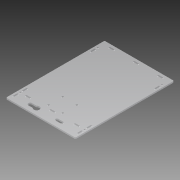
# Autodesk Inventor part: plastic_part_1
Saved by Autodesk Inventor 2013 (Build 170138000, 138)
## iProperties
Shininess: 20.0
Created: 2013-02-12
Part Number: plastic_part_1
Document SubType Name: Modeling
Designer: Noa Izumi
Material: Default
Density: 1 g/cm^3
Density: 0.0
Volumn: 0.0
Area: 0.0
PropertySet Name: Model Information
Control State: 0
Master: False
Checked Out: False
Author: Noa Izumi
Autodesk Inventor part; units mm, degrees
ref_plane "YZ Plane" through (0, 0, 0) normal (1, 0, 0) x (0, 1, 0)
ref_plane "XZ Plane" through (0, 0, 0) normal (0, 1, 0) x (-1, 0, 0)
ref_plane "XY Plane" through (0, 0, 0) normal (0, 0, 1) x (1, 0, 0)
sketch "Sketch1" plane through (0, 0, 0) normal (0, 0, 1) x (1, 0, 0)
  line L0 (0, 0) -> (148, 0)
  line L1 (148, 0) -> (148, 210)
  line L2 (148, 210) -> (0, 210)
  line L3 (0, 210) -> (0, 0)
  dimension "d0" = 148
  dimension "d1" = 210
  constraints: 8 end point, 2 parallel, 1 horizontal, 1 perpendicular
  measures "d0" distance of L0.start L0.end
  measures "d1" distance of L2.end L0.start
extrude "Extrusion1" add sketch "Sketch1" along normal blind 3
sketch "Sketch2" plane through (0, 0, 3) normal (0, 0, 1) x (1, 0, 0)
  line L0 (0, 0) -> (0, 210) projected
  line L1 (148, 0) -> (0, 0) projected
  line L2 (148, 210) -> (148, 0) projected
  line L3 (0, 210) -> (148, 210) projected
  line L4 (4, 185) -> (7, 185)
  line L5 (7, 185) -> (7, 175)
  line L6 (7, 175) -> (4, 175)
  line L7 (4, 175) -> (4, 185)
  line L8 (4, 40) -> (7, 40)
  line L9 (7, 40) -> (7, 30)
  line L10 (7, 30) -> (4, 30)
  line L11 (4, 30) -> (4, 40)
  line L12 (4, 20) -> (7, 20)
  line L13 (7, 20) -> (7, 10)
  line L14 (7, 10) -> (4, 10)
  line L15 (4, 10) -> (4, 20)
  line L16 (141, 185) -> (144, 185)
  line L17 (144, 185) -> (144, 175)
  line L18 (144, 175) -> (141, 175)
  line L19 (141, 175) -> (141, 185)
  line L20 (141, 40) -> (144, 40)
  line L21 (144, 40) -> (144, 30)
  line L22 (144, 30) -> (141, 30)
  line L23 (141, 30) -> (141, 40)
  line L24 (141, 20) -> (144, 20)
  line L25 (144, 20) -> (144, 10)
  line L26 (144, 10) -> (141, 10)
  line L27 (141, 10) -> (141, 20)
  dimension "d8" = 10
  dimension "d10" = 10
  dimension "d11" = 10
  dimension "d12" = 10
  dimension "d13" = 10
  dimension "d16" = 10
  dimension "d17" = 10
  dimension "d18" = 10
  dimension "d19" = 10
  dimension "d43" = 4
  dimension "d44" = 4
  dimension "d45" = 3
  dimension "d46" = 3
  dimension "d47" = 4
  dimension "d48" = 3
  dimension "d49" = 3
  dimension "d50" = 4
  dimension "d51" = 4
  dimension "d52" = 3
  dimension "d194" = 25
  dimension "d195" = 25
  constraints: 48 end point, 12 parallel, 6 horizontal, 6 perpendicular, 2 point on line
  measures "d8" distance of L6.end L4.start
  measures "d10" distance of L10.end L8.start
  measures "d11" distance between parallel lines of L12 L10
  measures "d12" distance of L14.end L12.start
  measures "d13" distance between parallel lines of L1 L14
  measures "d16" distance of L16.end L17.end
  measures "d17" distance of L20.end L21.end
  measures "d18" distance of L24.end L25.end
  measures "d19" distance between parallel lines of L24 L22
  measures "d43" distance between parallel lines of L2 L21
  measures "d44" distance between parallel lines of L2 L25
  measures "d45" distance of L20.start L20.end
  measures "d46" distance of L25.end L26.end
  measures "d47" distance between parallel lines of L2 L17
  measures "d48" distance of L16.start L16.end
  measures "d49" distance of L5.end L6.end
  measures "d50" distance between parallel lines of L0 L7
  measures "d51" distance between parallel lines of L0 L15
  measures "d52" distance of L9.end L10.end
  measures "d194" distance between parallel lines of L4 L3
  measures "d195" distance between parallel lines of L16 L3
extrude "Extrusion2" cut sketch "Sketch2" against normal through all contours L4 L5 L6 L7 | L8 L9 L10 L11 | L12 L13 L14 L15 | L16 L17 L18 L19 | L20 L21 L22 L23 | L24 L25 L26 L27
sketch "Sketch3" plane through (0, 0, 3) normal (0, 0, 1) x (1, 0, 0)
  line L0 (7, 30) -> (4, 30) projected
  line L1 (7, 20) -> (7, 10) projected
  line L2 (0, 210) -> (148, 210) projected
  line L3 (7, 185) -> (7, 175) projected
  line L4 (141, 175) -> (141, 185) projected
  point P0 (5.5, 190)
  point P1 (142.5, 190)
  point P2 (5.5, 25)
  point P3 (142.5, 25)
  point P4 (141, 30)
  dimension "d24" = 5
  dimension "d54" = 1.5
  dimension "d189" = 1.5
  dimension "d192" = 20
  dimension "d193" = 20
  dimension "d196" = 1.5
  dimension "d197" = 1.5
  measures "d24" distance from line of point (5.5, 25) L0
  measures "d54" horizontal distance of point (141, 30) point (142.5, 25)
  measures "d189" distance from line of L1 point (5.5, 25)
  measures "d192" distance from line of point (5.5, 190) L2
  measures "d193" distance from line of point (142.5, 190) L2
  measures "d196" distance from line of L3 point (5.5, 190)
  measures "d197" distance from line of L4 point (142.5, 190)
hole "Hole1" at (5.5, 190, 3) at (142.5, 190, 3) at (5.5, 25, 3) at (142.5, 25, 3) direction (0, 0, -1) diameter 3 end through all
fillet "Fillet1" radius 2 4 edges at (0, 0, 1.5) (148, 0, 1.5) (0, 210, 1.5) (148, 210, 1.5)
sketch "Sketch4" plane through (0, 0, 3) normal (0, 0, 1) x (1, 0, 0)
  line L0 (7, 20) -> (7, 10) projected
  line L1 (141, 10) -> (141, 20) projected
  line L2 (146, 0) -> (2, 0) projected
  line L3 (17, 26.5) -> (27, 26.5)
  line L4 (27, 26.5) -> (27, 23.5)
  line L5 (27, 23.5) -> (17, 23.5)
  line L6 (17, 23.5) -> (17, 26.5)
  line L7 (121, 23.5) -> (131, 23.5)
  line L8 (131, 23.5) -> (131, 26.5)
  line L9 (131, 26.5) -> (121, 26.5)
  line L10 (121, 26.5) -> (121, 23.5)
  line L11 (2, 210) -> (146, 210) projected
  line L12 (17, 204.5) -> (27, 204.5)
  line L13 (27, 204.5) -> (27, 201.5)
  line L14 (27, 201.5) -> (17, 201.5)
  line L15 (17, 201.5) -> (17, 204.5)
  line L16 (121, 204.5) -> (131, 204.5)
  line L17 (131, 204.5) -> (131, 201.5)
  line L18 (131, 201.5) -> (121, 201.5)
  line L19 (121, 201.5) -> (121, 204.5)
  line L20 (69, 26.5) -> (79, 26.5)
  line L21 (79, 26.5) -> (79, 23.5)
  line L22 (79, 23.5) -> (69, 23.5)
  line L23 (69, 23.5) -> (69, 26.5)
  line L24 (69, 204.5) -> (79, 204.5)
  line L25 (79, 204.5) -> (79, 201.5)
  line L26 (79, 201.5) -> (69, 201.5)
  line L27 (69, 201.5) -> (69, 204.5)
  line L28 (7, 185) -> (7, 175) projected
  line L29 (141, 175) -> (141, 185) projected
  dimension "d33" = 10
  dimension "d34" = 23.5
  dimension "d35" = 3
  dimension "d36" = 10
  dimension "d37" = 3
  dimension "d39" = 10
  dimension "d40" = 10
  dimension "d82" = 10
  dimension "d83" = 3
  dimension "d84" = 5.5
  dimension "d85" = 10
  dimension "d86" = 42
  dimension "d89" = 10
  dimension "d90" = 10
  dimension "d91" = 42
  dimension "d92" = 5.5
  dimension "d93" = 3
  dimension "d198" = 10
  dimension "d199" = 10
  constraints: 48 end point, 12 parallel, 6 horizontal, 6 perpendicular, 1 point on line
  measures "d33" distance of L4.end L5.end
  measures "d34" distance between parallel lines of L2 L5
  measures "d35" distance of L5.end L3.start
  measures "d36" distance of L7.start L7.end
  measures "d37" distance of L7.end L8.end
  measures "d39" distance between parallel lines of L6 L0
  measures "d40" distance between parallel lines of L1 L8
  measures "d82" distance of L12.start L12.end
  measures "d83" distance of L14.end L12.start
  measures "d84" distance between parallel lines of L11 L12
  measures "d85" distance of L21.end L22.end
  measures "d86" distance between parallel lines of L23 L4
  measures "d89" distance of L16.start L16.end
  measures "d90" distance of L24.start L24.end
  measures "d91" distance between parallel lines of L27 L13
  measures "d92" distance between parallel lines of L11 L16
  measures "d93" distance of L18.end L16.start
  measures "d198" distance from line of L14.end L28
  measures "d199" distance from line of L29 L16.end
extrude "Extrusion3" cut sketch "Sketch4" against normal through all
sketch "草圖15" plane through (0, 0, 3) normal (0, 0, 1) x (1, 0, 0)
  line L0 (0, 2) -> (0, 208) projected
  line L1 (146, 0) -> (2, 0) projected
  line L2 (148, 208) -> (148, 2) projected
  line L3 (95, 16.5) -> (105, 16.5)
  line L4 (108, 13.5) -> (108, 13.5)
  line L5 (105, 10.5) -> (95, 10.5)
  line L6 (92, 13.5) -> (92, 13.5)
  arc A0 (108, 13.5) -> (105, 16.5) centre (105, 13.5) ccw
  arc A1 (105, 10.5) -> (108, 13.5) centre (105, 13.5) ccw
  arc A2 (92, 13.5) -> (95, 10.5) centre (95, 13.5) ccw
  arc A3 (95, 16.5) -> (92, 13.5) centre (95, 13.5) ccw
  arc A4 (48.0314, 9) -> (48.0314, 18) centre (52, 13.5) ccw
  line L7 (38, 17.5) -> (46.7085, 17.5)
  line L8 (46.7085, 9.5) -> (38, 9.5)
  line L9 (34, 13.5) -> (34, 13.5)
  arc A5 (38, 17.5) -> (34, 13.5) centre (38, 13.5) ccw
  arc A6 (34, 13.5) -> (38, 9.5) centre (38, 13.5) ccw
  arc A7 (46.7085, 17.5) -> (48.0314, 18) centre (46.7085, 19.5) ccw
  arc A8 (48.0314, 9) -> (46.7085, 9.5) centre (46.7085, 7.5) ccw
  point P0 (0, 0)
  point P1 (92, 16.5)
  point P2 (108, 16.5)
  point P3 (92, 10.5)
  point P4 (34, 17.5)
  point P5 (34, 9.5)
  point P6 (47.5279, 17.5)
  point P7 (47.5279, 9.5)
  dimension "d159" = 16
  dimension "d161" = 6
  dimension "d163" = 40
  dimension "d164" = 3
  dimension "d165" = 12
  dimension "d166" = 13.5
  dimension "d167" = 13.5
  dimension "d168" = 52
  dimension "d169" = 8
  dimension "d173" = 4
  dimension "d174" = 2
  constraints: 20 point on circle, 16 tangent, 14 end point, 12 point on line, 9 centre point, 5 equal radius, 3 parallel, 2 horizontal, 1 perpendicular
  measures "d159" distance of point (92, 16.5) point (108, 16.5)
  measures "d161" distance of point (92, 10.5) point (92, 16.5)
  measures "d163" distance between parallel lines of L2 L4
  measures "d164" radius of A0
  measures "d165" diameter of A4
  measures "d166" distance from line of L1 A2.centre
  measures "d167" distance from line of L1 A4.centre
  measures "d168" distance from line of A4.centre L0
  measures "d169" distance of point (34, 9.5) point (34, 17.5)
  measures "d173" radius of A5
  measures "d174" radius of A7
extrude "擠出8" cut sketch "草圖15" against normal through all
sketch "草圖16" plane through (0, 0, 3) normal (0, 0, 1) x (1, 0, 0)
  line L0 (0, 2) -> (0, 208) projected
  line L1 (146, 0) -> (2, 0) projected
  point P0 (0, 0)
  point P1 (59, 32)
  point P2 (89, 32)
  point P3 (59, 62)
  point P4 (89, 62)
  dimension "d177" = 32
  dimension "d178" = 30
  dimension "d180" = 59
  dimension "d181" = 30
  measures "d177" distance from line of L1 point (59, 32)
  measures "d178" distance of point (89, 32) point (59, 32)
  measures "d180" distance from line of L0 point (59, 32)
  measures "d181" distance of point (59, 32) point (59, 62)
hole "孔7" at (59, 32, 3) at (89, 32, 3) at (59, 62, 3) at (89, 62, 3) direction (0, 0, -1) diameter 4 end through all
